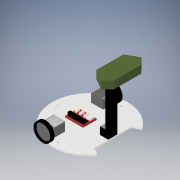
# Autodesk Inventor part: Top and middle round
Saved by Autodesk Inventor 2018 (Build 220112000, 112)
## iProperties
Created: 2018-10-22
Part Number: Top and middle round
Material: Generic
Document SubType Name: Modeling
Designer: Melda
Density: 1 g/cm^3
Appearance: White
Author: Melda
Autodesk Inventor part; units mm, degrees
ref_plane "YZ Plane" through (0, 0, 0) normal (1, 0, 0) x (0, 1, 0)
ref_plane "XZ Plane" through (0, 0, 0) normal (0, 1, 0) x (-1, 0, 0)
ref_plane "XY Plane" through (0, 0, 0) normal (0, 0, 1) x (1, 0, 0)
sketch "Sketch1" plane through (0, 0, 0) normal (0, 1, 0) x (-1, 0, 0)
  arc A0 (-99.8914, -75.1446) -> (-99.8914, 75.1446) centre (0, 0) ccw
  arc A1 (-99.8914, -75.1446) -> (-99.8914, 75.1446) centre (0, 0) ccw
  line L0 (-76.9728, 61.9125) -> (-99.8914, 75.1446)
  line L1 (-76.9728, -61.9125) -> (-99.8914, -75.1446)
  line L2 (-76.9728, -61.9125) -> (-76.9728, 61.9125)
  point P0 (-99.8914, -75.1446)
  dimension "d0" = 250
  dimension "d85" = 250
  constraints: 6 end point, 5 point on circle, 2 centre point, 2 coincident, 1 vertical
  measures "d0" diameter of A0
  measures "d85" diameter of A1
extrude "Extrusion1" add sketch "Sketch1" along normal blind 5
sketch "Sketch2" plane through (0, 5, 0) normal (0, 1, 0) x (1, 0, 0)
  circle A0 centre (-105, 0) radius 4
  circle A1 centre (0, 105) radius 4.3333
  circle A2 centre (0, -105) radius 4.3461
  arc A3 (99.8914, 75.1446) -> (99.8914, -75.1446) centre (0, 0) ccw
  dimension "d9" = 8
  dimension "d10" = 105
  dimension "d11" = 105
  dimension "d12" = 105
  constraints: 4 centre point, 2 point on circle
  measures "d9" diameter of A0
  measures "d10" distance of A3.centre A0.centre
  measures "d11" distance of A3.centre A1.centre
  measures "d12" distance of A3.centre A2.centre
extrude "Extrusion2" cut sketch "Sketch2" against normal blind 10
sketch "Sketch3" plane through (0, 5, 0) normal (0, 1, 0) x (1, 0, 0)
  line L0 (-12.4113, -103.9862) -> (-74.803, -103.9862)
  line L1 (-74.803, -103.9862) -> (-74.803, -126.1252)
  line L2 (-74.803, -126.1252) -> (-12.4113, -126.1252)
  line L3 (-12.4113, -126.1252) -> (-12.4113, -103.9862)
  line L4 (-12.4113, 103.9862) -> (-74.803, 103.9862)
  line L5 (-74.803, 103.9862) -> (-74.803, 126.1252)
  line L6 (-74.803, 126.1252) -> (-12.4113, 126.1252)
  line L7 (-12.4113, 126.1252) -> (-12.4113, 103.9862)
  point P0 (0, 0)
  constraints: 16 end point, 2 parallel, 1 horizontal, 1 perpendicular
extrude "Extrusion3" cut sketch "Sketch3" against normal blind 10
sketch "Sketch4" plane through (0, 5, 0) normal (0, 1, 0) x (1, 0, 0)
  line L0 (-60, -22.6667) -> (0, -22.6667)
  line L1 (0, -22.6667) -> (0, 22.3333)
  line L2 (0, 22.3333) -> (-60, 22.3333)
  line L3 (-60, 22.3333) -> (-60, -22.6667)
  point P0 (0, 0)
  dimension "d17" = 45
  dimension "d18" = 60
  dimension "d19" = 0
  constraints: 8 end point, 2 parallel, 1 horizontal, 1 perpendicular
  measures "d17" distance of L2.end L0.start
  measures "d18" distance of L1.end L2.end
  measures "d19" distance from line of L1 point (0, 0)
extrude "Extrusion4" add sketch "Sketch4" along normal blind 4
sketch "Sketch6" plane through (0, 9, 0) normal (0, 1, 0) x (1, 0, 0)
  line L0 (-55.4373, -18.0557) -> (-3.5957, -18.0557)
  line L1 (-3.5957, -18.0557) -> (-3.5957, 0)
  line L2 (-3.5957, 0) -> (-55.4373, 0)
  line L3 (-55.4373, 0) -> (-55.4373, -18.0557)
  point P0 (0, 0)
  constraints: 8 end point, 2 parallel, 1 horizontal, 1 perpendicular
extrude "Extrusion5" add sketch "Sketch6" along normal blind 12
chamfer "Chamfer1" distance 10 angle 45 1 edges at (-29.5165, 21, 0)
sketch "Sketch7" plane through (0, 9, 0) normal (0, 1, 0) x (1, 0, 0)
  line L0 (-55.2421, 4.3039) -> (-49.7854, 4.3039)
  line L1 (-49.7854, 4.3039) -> (-49.7854, 18.6092)
  line L2 (-49.7854, 18.6092) -> (-55.2421, 18.6092)
  line L3 (-55.2421, 18.6092) -> (-55.2421, 4.3039)
  line L4 (-40.6418, 4.3039) -> (-35.48, 4.3039)
  line L5 (-35.48, 4.3039) -> (-35.48, 18.6092)
  line L6 (-35.48, 18.6092) -> (-40.6418, 18.6092)
  line L7 (-40.6418, 18.6092) -> (-40.6418, 4.3039)
  line L8 (-26.3364, 4.3039) -> (-20.7323, 4.3039)
  line L9 (-20.7323, 4.3039) -> (-20.7323, 18.6092)
  line L10 (-20.7323, 18.6092) -> (-26.3364, 18.6092)
  line L11 (-26.3364, 18.6092) -> (-26.3364, 4.3039)
  line L12 (-4.0673, 4.3039) -> (-16.8978, 4.3039)
  line L13 (-16.8978, 4.3039) -> (-16.8978, 18.6092)
  line L14 (-16.8978, 18.6092) -> (-4.0673, 18.6092)
  line L15 (-4.0673, 18.6092) -> (-4.0673, 4.3039)
  point P0 (0, 0)
  constraints: 32 end point, 8 parallel, 6 point on line, 4 horizontal, 4 perpendicular
extrude "Extrusion6" add sketch "Sketch7" along normal blind 6
sketch "Sketch8" plane through (0, 5, 0) normal (0, 1, 0) x (1, 0, 0)
  line L0 (-59.1407, -97.913) -> (-19.1407, -97.913)
  line L1 (-19.1407, -97.913) -> (-19.1407, -62.913)
  line L2 (-19.1407, -62.913) -> (-59.1407, -62.913)
  line L3 (-59.1407, -62.913) -> (-59.1407, -97.913)
  line L4 (-59.1407, 97.913) -> (-19.1407, 97.913)
  line L5 (-19.1407, 97.913) -> (-19.1407, 62.913)
  line L6 (-19.1407, 62.913) -> (-59.1407, 62.913)
  line L7 (-59.1407, 62.913) -> (-59.1407, 97.913)
  point P0 (0, 0)
  dimension "d29" = 40
  dimension "d30" = 35
  constraints: 16 end point, 2 horizontal, 2 parallel, 1 perpendicular
  measures "d29" distance of L0.start L0.end
  measures "d30" distance of L2.end L0.start
extrude "Extrusion7" add sketch "Sketch8" along normal blind 30
fillet "Fillet1" radius 5 4 edges at (-59.1407, 35, 80.413) (-19.1407, 35, 80.413) (-59.1407, 35, -80.413) (-19.1407, 35, -80.413)
sketch "Sketch9" plane through (-59.1407, 5, 97.913) normal (0, 0, 1) x (1, 0, 0)
  line L0 (-10.2269, 0) -> (46.7294, 0) projected
  line L1 (5, 30) -> (35, 30) projected
  line L2 (40, 0) -> (40, 25) projected
  line L3 (0, 0) -> (0, 25) projected
  circle A0 centre (20, 15) radius 2.5
  point P0 (59.1407, -5)
  dimension "d34" = 30
  dimension "d35" = 15
  dimension "d36" = 40
  dimension "d37" = 20
  dimension "d38" = 5
  constraints: 1 centre point, 1 coincident
  measures "d34" distance between parallel lines of L0 L1
  measures "d35" distance from line of L1 point (20, 15)
  measures "d36" distance between parallel lines of L2 L3
  measures "d37" distance from line of L3 point (20, 15)
  measures "d38" diameter of A0
extrude "Extrusion8" add sketch "Sketch9" along normal blind 10
sketch "Sketch10" plane through (-19.1407, 5, -97.913) normal (0, 0, -1) x (-1, 0, 0)
  circle A0 centre (20, 15) radius 2.5 projected
  circle A1 centre (20, 15) radius 2.5
  point P0 (-19.1407, -5)
  constraints: 1 centre point, 1 coincident
extrude "Extrusion9" add sketch "Sketch10" along normal blind 10
sketch "Sketch11" plane through (0, 0, 0) normal (0, -1, 0) x (1, 0, 0)
  circle A0 centre (-39.1407, -84.5603) radius 2.5
  circle A1 centre (-39.1407, -84.5603) radius 2.375
  line L0 (65, -55) -> (65, 55) projected
  circle A2 centre (-39.1407, 84.5603) radius 2.5
  circle A3 centre (-39.1407, 84.5603) radius 2.375
  point P0 (0, 0)
  dimension "d43" = 5
  dimension "d44" = 4.75
  constraints: 4 centre point, 2 coincident
  measures "d43" diameter of A0
  measures "d44" diameter of A1
extrude "Extrusion10" cut sketch "Sketch11" against normal blind 2
fillet "Fillet2" radius 2 2 edges at (-41.5157, 0, 84.5603) (-41.5157, 0, -84.5603)
sketch "Sketch12" plane through (0, 0, 0) normal (0, -1, 0) x (1, 0, 0)
  circle A0 centre (45, 0) radius 5
  line L0 (65, -55) -> (65, 55) projected
  point P0 (0, 0)
  dimension "d50" = 10
  dimension "d51" = 20
  constraints: 1 centre point
  measures "d50" diameter of A0
  measures "d51" distance from line of L0 A0.centre
extrude "Extrusion11" add sketch "Sketch12" along normal blind 10
sketch "Sketch13" plane through (-39.1407, 20, -107.913) normal (0, 0, -1) x (-1, 0, 0)
  circle A0 centre (0, 0) radius 30
  point P0 (-39.1407, -20)
  dimension "d54" = 60
  constraints: 1 centre point
  measures "d54" diameter of A0
extrude "Extrusion12" add sketch "Sketch13" along normal blind 10
sketch "Sketch14" plane through (-39.1407, 20, -117.913) normal (0, 0, -1) x (-1, 0, 0)
  circle A0 centre (0, 0) radius 25
  point P0 (-39.1407, -20)
  dimension "d57" = 50
  constraints: 1 centre point
  measures "d57" diameter of A0
extrude "Extrusion13" cut sketch "Sketch14" against normal blind 5
sketch "Sketch16" plane through (-39.1407, 20, 107.913) normal (0, 0, 1) x (1, 0, 0)
  circle A0 centre (0, 0) radius 30
  point P0 (39.1407, -20)
  constraints: 1 centre point
extrude "Extrusion15" add sketch "Sketch16" along normal blind 10
sketch "Sketch17" plane through (-39.1407, 20, 117.913) normal (0, 0, 1) x (1, 0, 0)
  circle A0 centre (0, 0) radius 25
  point P0 (39.1407, -20)
  constraints: 1 centre point
extrude "Extrusion16" cut sketch "Sketch17" against normal blind 5
sketch "Sketch22" plane through (0, 5, 0) normal (0, 1, 0) x (1, 0, 0)
  line L0 (65.9728, -15) -> (75.9728, -15)
  line L1 (75.9728, -15) -> (75.9728, 15)
  line L2 (75.9728, 15) -> (65.9728, 15)
  line L3 (65.9728, 15) -> (65.9728, -15)
  line L4 (76.9728, -61.9125) -> (76.9728, 61.9125) projected
  point P0 (0, 0)
  dimension "d88" = 30
  dimension "d89" = 10
  dimension "d91" = 1
  dimension "d92" = 123.825
  dimension "d93" = 46.9125
  dimension "d94" = 46.9125
  constraints: 8 end point, 2 parallel, 1 horizontal, 1 perpendicular
  measures "d88" distance of L2.end L0.start
  measures "d89" distance of L1.end L2.end
  measures "d91" distance between parallel lines of L4 L1
  measures "d92" distance of L4.start L4.end
  measures "d93" distance from line of L4.end L2
  measures "d94" vertical distance of L4.start L0.end
extrude "Extrusion19" add sketch "Sketch22" along normal blind 210
sketch "Sketch23" plane through (65.9728, 5, -15) normal (-1, 0, 0) x (0, 0, 1)
  line L0 (-30, 210) -> (60, 210)
  line L1 (60, 210) -> (60, 190)
  line L2 (60, 190) -> (-30, 190)
  line L3 (-30, 190) -> (-30, 210)
  line L4 (30, 0) -> (30, 210) projected
  line L5 (0, 0) -> (0, 210) projected
  point P0 (15, -5)
  dimension "d97" = 20
  dimension "d98" = 90
  dimension "d99" = 30
  dimension "d100" = 30
  constraints: 8 end point, 2 parallel, 1 horizontal, 1 perpendicular
  measures "d97" distance of L0.end L1.end
  measures "d98" distance of L0.start L0.end
  measures "d99" distance between parallel lines of L4 L5
  measures "d100" distance between parallel lines of L4 L1
extrude "Extrusion20" add sketch "Sketch23" against normal blind 60
sketch "Sketch24" plane through (0, 5, 0) normal (0, 1, 0) x (1, 0, 0)
  line L0 (75.9728, -15) -> (65.9728, -15) projected
  line L1 (65.9728, -15) -> (49.2125, -15)
  line L2 (49.2125, -15) -> (49.2125, 15)
  line L3 (49.2125, 15) -> (65.9728, 15)
  line L4 (65.9728, 15) -> (65.9728, -15)
  point P0 (0, 0)
  constraints: 8 end point, 2 parallel, 1 horizontal, 1 perpendicular
extrude "Extrusion21" add sketch "Sketch24" along normal blind 25
sketch "Sketch25" plane through (0, 215, 0) normal (0, 1, 0) x (1, 0, 0)
  line L0 (65.9728, 45) -> (125.9728, 45) projected
  line L1 (65.9728, 45) -> (104.4639, 67.2228)
  line L2 (104.4639, 67.2228) -> (125.9728, 45)
  line L3 (65.9728, -45) -> (104.4639, -67.2228)
  line L4 (104.4639, -67.2228) -> (125.9728, -45)
  line L5 (65.9728, 45) -> (65.9728, -45) projected
  line L6 (65.9728, -45) -> (65.9728, 45)
  line L7 (125.9728, 45) -> (125.9728, -45) projected
  line L8 (125.9728, -45) -> (125.9728, 45)
  point P0 (0, 0)
  dimension "d105" = 30
  constraints: 12 end point, 1 collinear
  measures "d105" angle of L0 L1
extrude "Extrusion22" add sketch "Sketch25" against normal blind 25
body "Solid1"
